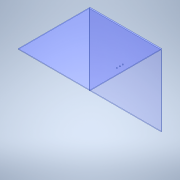
# Autodesk Inventor part: Frame Test for Papa John
Saved by Autodesk Inventor 2020 (Build 240168000, 168)
## iProperties
Created: 2020-02-02
Part Number: Frame Test for Papa John
Material: Generic
Document SubType Name: Modeling
Designer: aidan
Density: 1 g/cm^3
Appearance: Clear - Blue
Author: aidan
Autodesk Inventor part; units mm, degrees
ref_plane "YZ Plane" through (0, 0, 0) normal (1, 0, 0) x (0, 1, 0)
ref_plane "XZ Plane" through (0, 0, 0) normal (0, 1, 0) x (-1, 0, 0)
ref_plane "XY Plane" through (0, 0, 0) normal (0, 0, 1) x (1, 0, 0)
sketch "Sketch1" plane through (0, 0, 0) normal (0, 0, 1) x (1, 0, 0)
  line L0 (-169.6995, 150.4778) -> (135.1005, 150.4778)
  line L1 (135.1005, 150.4778) -> (135.1005, -154.3222)
  line L2 (135.1005, -154.3222) -> (-169.6995, -154.3222)
  line L3 (-169.6995, -154.3222) -> (-169.6995, 150.4778)
  point P0 (0, 0)
  dimension "d0" = 304.8
  constraints: 8 end point, 2 parallel, 2 perpendicular, 1 horizontal
  measures "d0" distance of L0.start L0.end
extrude "Extrusion1" add sketch "Sketch1" along normal blind 2.9972
sketch "Sketch2" plane through (0, 0, 2.9972) normal (0, 0, 1) x (1, 0, 0)
  line L0 (135.1005, 150.4778) -> (-169.6995, 150.4778) projected
  line L1 (135.1005, -154.3222) -> (135.1005, 150.4778) projected
  line L2 (-169.6995, 150.4778) -> (135.1005, 150.4778)
  line L3 (135.1005, 150.4778) -> (135.1005, 147.4806)
  line L4 (135.1005, 147.4806) -> (-169.6995, 147.4806)
  line L5 (-169.6995, 147.4806) -> (-169.6995, 150.4778)
  point P0 (0, 0)
  dimension "d3" = 2.9972
  constraints: 8 end point, 2 parallel, 1 horizontal, 1 perpendicular, 1 point on line
  measures "d3" distance of L4.end L0.end
extrude "Extrusion2" add sketch "Sketch2" along normal blind 301.8028
sketch "Sketch3" plane through (-169.6995, 150.4778, 0) normal (0, 1, 0) x (1, 0, 0)
  circle A0 centre (279.4, -139.7) radius 1.7272
  circle A1 centre (279.4, -152.4) radius 1.7272
  circle A2 centre (279.4, -165.1) radius 1.7272
  line L0 (279.4, -137.0931) -> (279.4, -150.7928) construction
  line L1 (304.8, 0) -> (304.8, -304.8) projected
  line L2 (304.8, -304.8) -> (0, -304.8) projected
  point P0 (169.6995, 0)
  dimension "d6" = 3.4544
  dimension "d7" = 12.7
  dimension "d8" = 12.7
  dimension "d9" = 25.4
  dimension "d10" = 152.4
  constraints: 3 centre point, 3 point on line, 2 end point, 2 equal radius, 1 vertical
  measures "d6" diameter of A0
  measures "d7" distance of A0.centre A1.centre
  measures "d8" distance of A1.centre A2.centre
  measures "d9" distance between parallel lines of L1 L0
  measures "d10" distance from line of L2 A1.centre
extrude "Extrusion3" cut sketch "Sketch3" against normal through all
body "Solid1"
